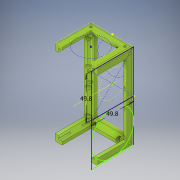
# Autodesk Inventor part: 10_Cube_2x1_v3
Saved by Autodesk Inventor 2019 (Build 230136000, 136)
## iProperties
Created: 2019-07-01
Part Number: 10_Cube_2x1_v3
Material: Generic
Document SubType Name: Modeling
Designer: diederichbenedict
Density: 1 g/cm^3
Appearance: IPHT_Grün
Author: diederichbenedict
Autodesk Inventor part; units mm, degrees
ref_plane "YZ Plane" through (0, 0, 0) normal (1, 0, 0) x (0, 1, 0)
ref_plane "XZ Plane" through (0, 0, 0) normal (0, 1, 0) x (-1, 0, 0)
sketch "Sketch1" plane through (0, 0, 0) normal (0, 0, 1) x (1, 0, 0)
  line L0 (-24.9, 49.9) -> (24.9, 49.9)
  line L1 (24.9, 49.9) -> (24.9, -49.9)
  line L2 (24.9, -49.9) -> (-24.9, -49.9)
  line L3 (-24.9, -49.9) -> (-24.9, 49.9)
  line L4 (-24.9, 49.9) -> (24.9, -49.9) construction
  line L5 (24.9, 49.9) -> (-24.9, -49.9) construction
  line L6 (16.9, 41.9) -> (-16.9, 41.9)
  line L7 (-16.9, 41.9) -> (-16.9, -41.9)
  line L8 (-16.9, -41.9) -> (16.9, -41.9)
  line L9 (16.9, -41.9) -> (16.9, 41.9)
  point P0 (0, 0)
  dimension "d0" = 49.8
  dimension "d1" = 99.8
  dimension "d2" = 8
  constraints: 20 end point, 4 parallel, 2 midpoint, 2 perpendicular, 1 horizontal, 3 other
  measures "d0" distance of L1.end L2.end
  measures "d1" distance of L0.end L1.end
  measures "d2" distance between parallel lines of L0 L6
extrude "Extrusion1" add sketch "Sketch1" along normal blind 8
sketch "Sketch2" plane through (0, 0, 8) normal (0, 0, 1) x (1, 0, 0)
  line L0 (16.9, 41.9) -> (16.9, -41.9) projected
  line L1 (16.9, -41.9) -> (-16.9, -41.9) projected
  line L2 (-16.9, -41.9) -> (-16.9, 41.9) projected
  line L3 (-16.9, 41.9) -> (16.9, 41.9) projected
  line L4 (24.9, 49.9) -> (-24.9, 49.9) projected
  line L5 (-24.9, 49.9) -> (-24.9, -49.9) projected
  line L6 (-24.9, -49.9) -> (24.9, -49.9) projected
  line L7 (24.9, -49.9) -> (24.9, 49.9) projected
  line L8 (16.9, -41.9) -> (24.9, -41.9)
  line L9 (24.9, -41.9) -> (24.9, -49.9)
  line L10 (24.9, -49.9) -> (16.9, -49.9)
  line L11 (16.9, -49.9) -> (16.9, -41.9)
  line L12 (16.9, 41.9) -> (-16.9, 41.9) projected
  line L13 (24.9, 49.9) -> (16.9, 49.9)
  line L14 (16.9, 49.9) -> (16.9, 41.9)
  line L15 (16.9, 41.9) -> (24.9, 41.9)
  line L16 (24.9, 41.9) -> (24.9, 49.9)
  line L17 (-24.9, -49.9) -> (-16.9, -49.9)
  line L18 (-16.9, -49.9) -> (-16.9, -41.9)
  line L19 (-16.9, -41.9) -> (-24.9, -41.9)
  line L20 (-24.9, -41.9) -> (-24.9, -49.9)
  line L21 (-24.9, 49.9) -> (-16.9, 49.9)
  line L22 (-16.9, 49.9) -> (-16.9, 41.9)
  line L23 (-16.9, 41.9) -> (-24.9, 41.9)
  line L24 (-24.9, 41.9) -> (-24.9, 49.9)
  point P0 (0, 0)
  constraints: 32 end point, 8 parallel, 4 horizontal, 4 perpendicular
extrude "Extrusion2" add sketch "Sketch2" along normal blind 33.8 contours L14 L4 L7 L15 | L8 L7 L6 L11 | L23 L5 L4 L22 | L18 L6 L5 L19
sketch "Sketch3" plane through (0, 0, 0) normal (0, 0, -1) x (-1, 0, 0)
  line L0 (24.9, -49.9) -> (24.9, 49.9) construction
  line L1 (24.9, 49.9) -> (-24.9, 49.9) construction
  line L2 (-24.9, -49.9) -> (24.9, -49.9) construction
  line L3 (-24.9, 49.9) -> (-24.9, -49.9) construction
  line L4 (-19.9, -44.9) -> (20.1, -44.9) construction
  line L5 (20.1, -44.9) -> (20.1, -4.9) construction
  line L6 (20.1, -4.9) -> (-19.9, -4.9) construction
  line L7 (-19.9, -4.9) -> (-19.9, -44.9) construction
  line L8 (-19.9, 44.9) -> (20.1, 44.9) construction
  line L9 (20.1, 44.9) -> (20.1, 4.9) construction
  line L10 (20.1, 4.9) -> (-19.9, 4.9) construction
  line L11 (-19.9, 4.9) -> (-19.9, 44.9) construction
  point P0 (19.9, 44.9)
  point P1 (19.9, -44.9)
  dimension "d95" = 5
  dimension "d96" = 5
  dimension "d97" = 5
  dimension "d98" = 5
  dimension "d99" = 5
  dimension "d100" = 5
  dimension "d101" = 5
  dimension "d102" = 5
  dimension "d115" = 40
  dimension "d116" = 40
  dimension "d117" = 40
  dimension "d118" = 40
  constraints: 16 end point, 4 parallel, 2 horizontal, 2 perpendicular
  measures "d95" distance from line of L1 point (19.9, 44.9)
  measures "d96" distance from line of point (19.9, 44.9) L0
  measures "d97" distance from line of point (19.9, -44.9) L0
  measures "d98" distance from line of point (19.9, -44.9) L2
  measures "d99" distance from line of L4.start L2
  measures "d100" distance from line of L4.start L3
  measures "d101" distance from line of L8.start L3
  measures "d102" distance from line of L8.start L1
  measures "d115" distance of L6.end L5.end
  measures "d116" distance of L5.end L4.end
  measures "d117" distance of L9.end L10.end
  measures "d118" distance of L8.end L9.end
hole "Hole1" at (-19.9, 44.9, 0) at (-19.9, -44.9, 0) at (19.9, -44.9, 0) at (19.9, 44.9, 0) at (19.9, -4.9, 0) at (19.9, 4.9, 0) at (-20.1, -4.9, 0) at (-20.1, 4.9, 0) direction (0, 0, 1) diameter 2.8 depth 16 tip angle 118 counterbore diameter 5.5 counterbore depth 3.1
sketch "Sketch4" plane through (-24.9, 49.9, 0) normal (0, 1, 0) x (1, 0, 0)
  line L0 (0, 0) -> (49.8, 0) construction
  line L1 (0, 0) -> (0, -41.8) construction
  line L2 (8, -41.8) -> (0, -41.8) construction
  line L3 (8, -8) -> (8, -41.8) construction
  line L4 (41.8, -8) -> (8, -8) construction
  line L5 (41.8, -8) -> (41.8, -41.8) construction
  line L6 (49.8, -41.8) -> (41.8, -41.8) construction
  line L7 (49.8, 0) -> (49.8, -41.8) construction
  circle A0 centre (24.9, -24.9) radius 16.9 construction
  point P0 (24.9, 0)
  constraints: 3 tangent, 1 centre point
sketch "Sketch5" plane through (0, 0, 0) normal (0, 0, -1) x (-1, 0, 0)
  line L0 (-16.9, -41.9) -> (-16.9, 41.9) construction
  line L1 (-16.9, 41.9) -> (16.9, 41.9) construction
  line L2 (16.9, 41.9) -> (16.9, -41.9) construction
  line L3 (16.9, -41.9) -> (-16.9, -41.9) construction
  circle A0 centre (0, 25) radius 16.9 construction
  point P0 (0, 0)
  constraints: 3 tangent, 1 centre point
fillet "Fillet1" radius 2 8 edges at (24.9, 49.9, 20.9) (24.9, -49.9, 20.9) (-24.9, -49.9, 20.9) (-24.9, 49.9, 20.9) (-24.9, 0, 0) (0, -49.9, 0) (24.9, 0, 0) (0, 49.9, 0)
sketch "Sketch6" plane through (0, 0, 41.8) normal (0, 0, 1) x (1, 0, 0)
  arc A0 (-22.9, 49.9) -> (-24.9, 47.9) centre (-22.9, 47.9) ccw projected
  line L0 (-24.9, 47.9) -> (-24.9, 41.9) projected
  line L1 (-24.9, 41.9) -> (-16.9, 41.9) projected
  line L2 (-16.9, 41.9) -> (-16.9, 49.9) projected
  line L3 (-16.9, 49.9) -> (-22.9, 49.9) projected
  arc A1 (24.9, 47.9) -> (22.9, 49.9) centre (22.9, 47.9) ccw projected
  line L4 (22.9, 49.9) -> (16.9, 49.9) projected
  line L5 (16.9, 49.9) -> (16.9, 41.9) projected
  line L6 (16.9, 41.9) -> (24.9, 41.9) projected
  line L7 (24.9, 41.9) -> (24.9, 47.9) projected
  arc A2 (22.9, -49.9) -> (24.9, -47.9) centre (22.9, -47.9) ccw projected
  line L8 (24.9, -47.9) -> (24.9, -41.9) projected
  line L9 (24.9, -41.9) -> (16.9, -41.9) projected
  line L10 (16.9, -41.9) -> (16.9, -49.9) projected
  line L11 (16.9, -49.9) -> (22.9, -49.9) projected
  arc A3 (-24.9, -47.9) -> (-22.9, -49.9) centre (-22.9, -47.9) ccw projected
  line L12 (-22.9, -49.9) -> (-16.9, -49.9) projected
  line L13 (-16.9, -49.9) -> (-16.9, -41.9) projected
  line L14 (-16.9, -41.9) -> (-24.9, -41.9) projected
  line L15 (-24.9, -41.9) -> (-24.9, -47.9) projected
  line L16 (0, 38.1838) -> (54, 38.1838) construction
  line L17 (21.2838, 41.9) -> (16.9, 46.2838)
  line L18 (16.9, 49.9) -> (16.9, 41.9) projected
  line L19 (16.9, 46.2838) -> (16.9, 41.9)
  line L20 (16.9, 41.9) -> (21.2838, 41.9)
  line L21 (-16.9, 49.9) -> (-16.9, 41.9) projected
  line L22 (-16.9, 41.9) -> (-16.9, 46.2838)
  line L23 (-16.9, 46.2838) -> (-21.2838, 41.9)
  line L24 (-16.9, 46.2838) -> (-10.7004, 46.2838) construction
  line L25 (-16.9, -41.9) -> (-16.9, 41.9) projected
  line L26 (-21.2838, 41.9) -> (-16.9, 41.9)
  line L27 (-16.9, 41.9) -> (-21.2838, 41.9)
  line L28 (16.9, -41.9) -> (16.9, -49.9) projected
  line L29 (16.9, -41.9) -> (21.2838, -41.9)
  line L30 (24.9, -41.9) -> (16.9, -41.9) projected
  line L31 (21.2838, -41.9) -> (16.9, -46.2838)
  line L32 (16.9, -41.9) -> (16.9, -46.2838)
  line L33 (-16.9, -41.9) -> (-21.2838, -41.9)
  line L34 (-16.9, -41.9) -> (-16.9, -49.9) projected
  line L35 (-16.9, -41.9) -> (-16.9, -46.2838)
  line L36 (-21.2838, -41.9) -> (-16.9, -46.2838)
  dimension "d105" = 4.3838
  dimension "d106" = 4.3838
  dimension "d107" = 4.3838
  dimension "d108" = 4.3838
  dimension "d109" = 4.3838
  dimension "d110" = 4.3838
  dimension "d111" = 0
  constraints: 30 end point, 9 point on line, 3 collinear, 2 horizontal, 2 perpendicular, 1 equal length, 1 parallel, 1 vertical
  measures "d105" distance of L5.end L17.end
  measures "d106" distance of L5.end L17.start
  measures "d107" distance of L1.end L22.end
  measures "d108" distance of L23.end L1.end
  measures "d109" distance of L35.end L13.end
  measures "d110" distance of L33.end L13.end
  measures "d111" vertical distance of L35.end L31.end
extrude "Extrusion3" cut sketch "Sketch6" against normal up to surface (33.8 mm away) contours L13 L36 L14 | L2 L1 L23 | L6 L5 L17 | L10 L9 L31
sketch "Sketch7" plane through (-24.9, 41.9, 8) normal (0, -1, 0) x (1, 0, 0)
  line L0 (41.8, -8) -> (41.8, 0) construction
  line L1 (8, -8) -> (8, 0) construction
  line L2 (0, 0) -> (8, 0) construction
  line L3 (41.8, 33.8) -> (41.8, 0) construction
  line L4 (41.8, 0) -> (8, 0) construction
  circle A0 centre (24.9, 16.9) radius 16.9 construction
  line L5 (24.9, 54.9423) -> (-13.1423, 16.9) construction
  line L6 (-13.1423, 16.9) -> (24.9, -21.1423) construction
  line L7 (24.9, -21.1423) -> (62.9423, 16.9) construction
  line L8 (62.9423, 16.9) -> (24.9, 54.9423) construction
  line L9 (24.9, 54.9423) -> (24.9, -21.1423) construction
  line L10 (-13.1423, 16.9) -> (62.9423, 16.9) construction
  line L11 (24.9, 54.9423) -> (78.7, 54.9423) construction
  line L12 (41.8, 0) -> (41.8, 33.8) projected
  line L13 (41.8, 0) -> (41.8, -4.2423)
  line L14 (8, -4.2423) -> (8, 0)
  line L15 (41.8, -4.2423) -> (46.0423, 0)
  line L16 (44.5637, 0) -> (46.1838, 0) projected
  line L17 (41.8, 0) -> (46.0423, 0)
  line L18 (8, 33.8) -> (8, 0) projected
  line L19 (8, 0) -> (3.7577, 0)
  line L20 (3.6162, 0) -> (5.2363, 0) projected
  line L21 (3.7577, 0) -> (8, -4.2423)
  dimension "d37" = 53.8
  dimension "d38" = 135
  dimension "d39" = 53.8
  constraints: 26 end point, 8 point on line, 2 collinear, 2 horizontal, 2 midpoint, 2 parallel, 2 tangent, 1 centre point, 1 equal length, 1 perpendicular, 1 vertical
  measures "d37" distance of L5.start L5.end
  measures "d38" angle of L5 L11
  measures "d39" distance of L6.end L5.end
extrude "Extrusion4" cut sketch "Sketch7" along normal up to surface (83.8 mm away)
sketch "Sketch8" plane through (16.9, -49.9, 8) normal (-1, 0, 0) x (0, 0, 1)
  line L0 (8, 3.6) -> (-1.65, 3.6) construction
  line L1 (-4.2423, 8.1) -> (-4.2423, 41.9) construction
  line L2 (-4.2423, 8.1) -> (0, 3.7162) construction
  line L3 (0, 3.6162) -> (0, 0) projected
  line L4 (0, 3.6162) -> (-4.3838, 8)
  line L5 (-8, 8) -> (-4.2423, 8) projected
  line L6 (0, 3.6162) -> (6.1996, 3.6162) construction
  line L7 (0, 6.3799) -> (0, 8) projected
  line L8 (-4.3838, 8) -> (0, 8)
  line L9 (0, 8) -> (0, 3.6162)
  line L10 (0, 91.8) -> (-4.3838, 91.8)
  line L11 (0, 91.8) -> (-4.2423, 91.8) projected
  line L12 (-4.3838, 91.8) -> (0, 96.1838)
  line L13 (0, 96.1838) -> (0, 91.8)
  dimension "d121" = 135
  dimension "d122" = 45
  constraints: 20 end point, 3 perpendicular, 2 horizontal, 2 point on line, 1 collinear, 1 equal length, 1 vertical, 6 other
  measures "d121" angle of L6 L4
  measures "d122" angle of L10 L12
ref_plane "Work Plane1" through (-20.32, -18.034, 19.8181) normal (-1, 0, 0) x (0, 0, 1)
extrude "Extrusion5" cut sketch "Sketch8" along normal up to surface (33.8 mm away)
sketch "Sketch9" plane through (0, 0, 41.8) normal (0, 0, 1) x (1, 0, 0)
  arc A0 (19.6637, 43.5201) -> (18.5201, 44.6637) centre (19.9, 44.9) ccw projected
  arc A1 (18.5201, -44.6637) -> (19.6637, -43.5201) centre (19.9, -44.9) ccw projected
  arc A2 (-19.6637, -43.5201) -> (-18.5201, -44.6637) centre (-19.9, -44.9) ccw projected
  arc A3 (-18.5201, 44.6637) -> (-19.6637, 43.5201) centre (-19.9, 44.9) ccw projected
hole "Hole2" at (19.9, 44.9, 41.8) at (-19.9, 44.9, 41.8) at (19.9, -44.9, 41.8) at (-19.9, -44.9, 41.8) direction (0, 0, -1) diameter 2.8 depth 12 tip angle 118
sketch "Sketch11" plane through (24.9, -41.9, 8) normal (1, 0, 0) x (0, 0, -1)
  line L0 (-33.8, 89.8) -> (6, 89.8) construction
  line L1 (-33.8, 83.8) -> (-33.8, 89.8) construction
  line L2 (0, 83.8) -> (-33.8, 83.8) construction
  line L3 (0, 0) -> (0, 83.8) construction
  line L4 (0, 0) -> (-33.8, 0) construction
  line L5 (-33.8, -6) -> (-33.8, 0) construction
  line L6 (6, -6) -> (-33.8, -6) construction
  line L7 (6, 89.8) -> (6, -6) construction
  line L8 (-33.8, -8) -> (6, -8) construction
  line L9 (8, -6) -> (8, 89.8) construction
  line L10 (8, 91.8) -> (-33.8, 91.8) construction
  line L11 (-33.8, -3) -> (3, -3) construction
  line L12 (3, -3) -> (3, 86.8) construction
  line L13 (3, 86.8) -> (-33.8, 86.8) construction
  line L14 (-33.8, 86.8) -> (-33.8, -3) construction
  line L15 (3, 86.8) -> (3, 46.8) construction
  line L16 (3, -3) -> (3, 37) construction
  point P0 (3.1, -3.1)
  point P1 (3.1, 36.9)
  point P2 (8, 22.6681)
  point P3 (8, 61.1319)
  dimension "d88" = 5
  dimension "d89" = 5
  dimension "d90" = 5
  dimension "d113" = 40
  dimension "d114" = 40
  constraints: 12 end point, 2 parallel, 2 point on line, 1 horizontal, 1 midpoint, 1 perpendicular
  measures "d88" distance from line of L11.end L8
  measures "d89" distance between parallel lines of L10 L13
  measures "d90" distance between parallel lines of L9 L12
  measures "d113" distance of L12.end L15.end
  measures "d114" distance of L11.end L16.end
hole "Hole4" at (24.9, 44.9, 5) at (24.9, -44.9, 5) at (24.9, 4.9, 5) at (24.9, -5, 4.9) direction (-1, 0, 0) diameter 2.9 depth 6.5 tip angle 118
sketch "Sketch12" plane through (-16.9, -49.9, 8) normal (0, -1, 0) x (1, 0, 0)
  line L0 (-8, 33.8) -> (-8, -6) construction
  line L1 (-6, -8) -> (39.8, -8) construction
  line L2 (41.8, -6) -> (41.8, 33.8) construction
  line L3 (-6, -8) -> (39.8, -8) construction
  point P0 (-2.3319, -8)
  point P1 (36.1319, -8)
  point P2 (-3, -3)
  point P3 (36.8, -3)
  point P4 (37.6681, -8)
  dimension "d91" = 5
  dimension "d92" = 5
  dimension "d93" = 5
  dimension "d94" = 5
  measures "d91" distance from line of point (-3, -3) L0
  measures "d92" distance from line of point (-3, -3) L1
  measures "d93" distance from line of L3 point (36.8, -3)
  measures "d94" distance from line of L2 point (36.8, -3)
hole "Hole5" at (-19.9, -49.9, 5) at (19.9, -49.9, 5) direction (0, 1, 0) diameter 2.9 depth 6.5 tip angle 118
sketch "Sketch13" plane through (-24.9, -41.9, 8) normal (-1, 0, 0) x (0, 0, 1)
  circle A0 centre (-3, 86.8) radius 1.45 projected
  circle A1 centre (-3, -3) radius 1.45 projected
  arc A2 (-2.7907, 45.3652) -> (-2.7907, 48.2348) centre (-3, 46.8) ccw projected
  arc A3 (-2.7907, 35.4834) -> (-2.7907, 38.3166) centre (-3.1, 36.9) ccw projected
hole "Hole6" at (-24.9, 44.9, 5) at (-24.9, -44.9, 5) at (-24.9, 4.9, 5) at (-24.9, -5, 4.9) direction (1, 0, 0) diameter 2.9 depth 6.5 tip angle 118
sketch "Sketch14" plane through (-16.9, 49.9, 8) normal (0, 1, 0) x (1, 0, 0)
  circle A0 centre (36.8, 3) radius 1.45 projected
  circle A1 centre (-3, 3) radius 1.45 projected
hole "Hole7" at (-19.9, 49.9, 5) at (19.9, 49.9, 5) direction (0, -1, 0) diameter 2.9 depth 6.5 tip angle 118
sketch "Sketch15" plane through (24.9, -41.9, 8) normal (1, 0, 0) x (0, 0, -1)
  line L0 (8, 91.8) -> (-33.8, 91.8) construction
  line L1 (8, -6) -> (8, 89.8) projected
  line L2 (8, 91.8) -> (-41.8, 91.8)
  line L3 (-41.8, 91.8) -> (-41.8, 42)
  line L4 (-41.8, 42) -> (8, 42)
  line L5 (8, 42) -> (8, 91.8)
  line L6 (-41.8, 61.8634) -> (-41.8, 52.9) projected
  line L7 (8, 91.8) -> (-41.8, 42) construction
  line L8 (8, 42) -> (-41.8, 91.8) construction
  circle A0 centre (-16.9, 66.9) radius 15.6444 construction
  line L9 (-41.8, 42) -> (8, 42)
  line L10 (8, 42) -> (8, -7.8)
  line L11 (8, -7.8) -> (-41.8, -7.8)
  line L12 (-41.8, -7.8) -> (-41.8, 42)
  circle A1 centre (-16.9, 17.1) radius 24.9
  point P0 (8, 41.9)
  dimension "d119" = 49.8
  dimension "d120" = 49.8
  constraints: 20 end point, 4 parallel, 3 perpendicular, 3 tangent, 2 centre point, 2 horizontal, 1 midpoint, 1 point on line
  measures "d119" distance of L4.end L3.end
  measures "d120" distance of L3.end L2.end
sketch "Sketch16" plane through (0, 0, 0) normal (0, 0, -1) x (-1, 0, 0)
  arc A0 (-15.4548, 47.8) -> (-13.3452, 47.8) centre (-14.4, 45.7) ccw
  line L0 (-22.8, 47.8) -> (-15.4548, 47.8)
  line L1 (-22.8, 40.4548) -> (-22.8, 47.8)
  arc A1 (-22.8, 38.3452) -> (-22.8, 40.4548) centre (-20.7, 39.4) ccw
  line L2 (-22.8, 11.4548) -> (-22.8, 38.3452)
  arc A2 (-22.8, 9.3452) -> (-22.8, 11.4548) centre (-20.7, 10.4) ccw
  line L3 (-22.8, 2) -> (-22.8, 9.3452)
  line L4 (-15.4548, 2) -> (-22.8, 2)
  arc A3 (-13.3452, 2) -> (-15.4548, 2) centre (-14.4, 4.1) ccw
  line L5 (13.5452, 2) -> (-13.3452, 2)
  arc A4 (15.6548, 2) -> (13.5452, 2) centre (14.6, 4.1) ccw
  line L6 (23, 2) -> (15.6548, 2)
  line L7 (23, 9.3452) -> (23, 2)
  arc A5 (23, 11.4548) -> (23, 9.3452) centre (20.9, 10.4) ccw
  line L8 (23, 38.3452) -> (23, 11.4548)
  arc A6 (23, 40.4548) -> (23, 38.3452) centre (20.9, 39.4) ccw
  line L9 (23, 47.8) -> (23, 40.4548)
  line L10 (15.6548, 47.8) -> (23, 47.8)
  arc A7 (13.5452, 47.8) -> (15.6548, 47.8) centre (14.6, 45.7) ccw
  line L11 (-13.3452, 47.8) -> (13.5452, 47.8)
  circle A8 centre (-19.9, 4.9) radius 2.75
  circle A9 centre (20.1, 44.9) radius 2.75
  circle A10 centre (20.1, 4.9) radius 2.75
  circle A11 centre (-19.9, 44.9) radius 2.75
  line L12 (-16.8, 8) -> (-16.8, 41.8)
  line L13 (-16.8, 41.8) -> (17, 41.8)
  line L14 (17, 41.8) -> (17, 8)
  line L15 (17, 8) -> (-16.8, 8)
  line L16 (-16.9, -41.9) -> (-16.9, 41.9) construction
  line L17 (-16.9, 41.9) -> (16.9, 41.9) construction
  line L18 (16.9, 41.9) -> (16.9, -41.9) construction
  line L19 (16.9, -41.9) -> (-16.9, -41.9) construction
  circle A12 centre (20.1, 4.9) radius 2.75 construction
  circle A13 centre (-19.9, 4.9) radius 2.75 construction
  circle A14 centre (-19.9, 44.9) radius 2.75 construction
  circle A15 centre (19.9, -44.9) radius 2.75 construction
  circle A16 centre (19.9, 44.9) radius 2.75 construction
  circle A17 centre (-19.9, -44.9) radius 2.75 construction
  circle A18 centre (-19.9, -4.9) radius 2.75 construction
  circle A19 centre (20.1, -4.9) radius 2.75 construction
  line L20 (-22.9, 47.9) -> (22.9, 47.9) construction
  line L21 (-22.9, -47.9) -> (-22.9, 47.9) construction
  line L22 (22.9, -47.9) -> (-22.9, -47.9) construction
  line L23 (22.9, 47.9) -> (22.9, -47.9) construction
  arc A20 (-15.4548, -2) -> (-13.3452, -2) centre (-14.4, -4.1) ccw
  line L24 (-22.8, -2) -> (-15.4548, -2)
  line L25 (-22.8, -9.3452) -> (-22.8, -2)
  arc A21 (-22.8, -11.4548) -> (-22.8, -9.3452) centre (-20.7, -10.4) ccw
  line L26 (-22.8, -38.3452) -> (-22.8, -11.4548)
  arc A22 (-22.8, -40.4548) -> (-22.8, -38.3452) centre (-20.7, -39.4) ccw
  line L27 (-22.8, -47.8) -> (-22.8, -40.4548)
  line L28 (-15.4548, -47.8) -> (-22.8, -47.8)
  arc A23 (-13.3452, -47.8) -> (-15.4548, -47.8) centre (-14.4, -45.7) ccw
  line L29 (13.5452, -47.8) -> (-13.3452, -47.8)
  arc A24 (15.6548, -47.8) -> (13.5452, -47.8) centre (14.6, -45.7) ccw
  line L30 (23, -47.8) -> (15.6548, -47.8)
  line L31 (23, -40.4548) -> (23, -47.8)
  arc A25 (23, -38.3452) -> (23, -40.4548) centre (20.9, -39.4) ccw
  line L32 (23, -11.4548) -> (23, -38.3452)
  arc A26 (23, -9.3452) -> (23, -11.4548) centre (20.9, -10.4) ccw
  line L33 (23, -2) -> (23, -9.3452)
  line L34 (15.6548, -2) -> (23, -2)
  arc A27 (13.5452, -2) -> (15.6548, -2) centre (14.6, -4.1) ccw
  line L35 (-13.3452, -2) -> (13.5452, -2)
  circle A28 centre (-19.9, -44.9) radius 2.75
  circle A29 centre (20.1, -4.9) radius 2.75
  circle A30 centre (20.1, -44.9) radius 2.75
  circle A31 centre (-19.9, -4.9) radius 2.75
  line L36 (-16.8, -41.8) -> (-16.8, -8)
  line L37 (-16.8, -8) -> (17, -8)
  line L38 (17, -8) -> (17, -41.8)
  line L39 (17, -41.8) -> (-16.8, -41.8)
  point P0 (0, 0)
  point P1 (0.1, 24.9)
  point P2 (0.1, -24.9)
  constraints: 64 end point, 32 point on circle, 24 centre point
hole "Hole8" at (14.4, 45.7, 0) at (-14.6, 45.7, 0) at (-20.9, 39.4, 0) at (20.7, 39.4, 0) at (20.7, 10.4, 0) at (-20.9, 10.4, 0) at (-20.9, -10.4, 0) at (20.7, -10.4, 0) at (20.7, -39.4, 0) at (14.4, -45.7, 0) at (-14.6, -45.7, 0) at (-20.9, -39.4, 0) direction (0, 0, 1) diameter 4.7 end through all
body "Solid1"
